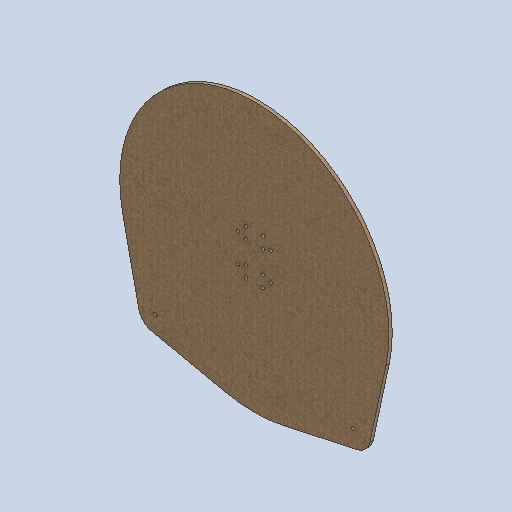
# Autodesk Inventor part: belt_liner_v1_MDF_throw_plate
Saved by Autodesk Inventor 2025.1 (Build 291241000, 241)
## iProperties
Created: 2024-12-08
Part Number: belt_liner_v1_MDF_throw_plate
Material: MDF 中密度繊維ボード
Document SubType Name: Modeling
Designer: haruy
Density: 0.8 g/cm^3
Appearance: ダンボール - 段ボール紙
Author: haruy
Autodesk Inventor part; units mm, degrees
ref_plane "YZ Plane" through (0, 0, 0) normal (1, 0, 0) x (0, 1, 0)
ref_plane "XZ Plane" through (0, 0, 0) normal (0, 1, 0) x (-1, 0, 0)
ref_plane "XY Plane" through (0, 0, 0) normal (0, 0, 1) x (1, 0, 0)
derived "belt_liner_v1_Sketch_Base.ipt"
sketch "スケッチ2" plane through (0, 0, 300) normal (0, 0, 1) x (1, 0, 0)
  circle A0 centre (0, 0) radius 120 projected
  circle A1 centre (-88.3883, -88.3883) radius 5 projected
  circle A2 centre (88.3883, -88.3883) radius 5 projected
  line L0 (0, 0) -> (0, -186.3039) projected
  line L1 (-10, 30) -> (10, 30) projected
  line L2 (10, 30) -> (10, -30) projected
  line L3 (10, -30) -> (-10, -30) projected
  line L4 (-10, -30) -> (-10, 30) projected
  line L5 (12, 2.5) -> (17, 2.5) projected
  line L6 (17, 2.5) -> (17, -2.5) projected
  line L7 (17, -2.5) -> (12, -2.5) projected
  line L8 (12, -2.5) -> (12, 2.5) projected
  circle A3 centre (-88.3883, -88.3883) radius 15 projected
  circle A4 centre (88.3883, -88.3883) radius 15 projected
  circle A5 centre (-7.5, -20) radius 1.5 projected
  circle A6 centre (-7.5, -10) radius 1.5 projected
  circle A7 centre (7.5, -10) radius 1.5 projected
  circle A8 centre (7.5, -20) radius 1.5 projected
  line L9 (0, 0) -> (10, 0) projected
  circle A9 centre (-7.5, 10) radius 1.5 projected
  circle A10 centre (-7.5, 20) radius 1.5 projected
  circle A11 centre (7.5, 10) radius 1.5 projected
  circle A12 centre (7.5, 20) radius 1.5 projected
  line L10 (12, 2.5) -> (17, 2.5) projected
  line L11 (17, 2.5) -> (17, 22.5) projected
  line L12 (17, 22.5) -> (12, 22.5) projected
  line L13 (12, 22.5) -> (12, 2.5) projected
  line L14 (12, -2.5) -> (17, -2.5) projected
  line L15 (17, -2.5) -> (17, -22.5) projected
  line L16 (17, -22.5) -> (12, -22.5) projected
  line L17 (12, -22.5) -> (12, -2.5) projected
  circle A13 centre (14.5, 12.5) radius 1.5 projected
  circle A14 centre (14.5, -12.5) radius 1.5 projected
  circle A15 centre (-14.5, 12.5) radius 1.5 projected
  circle A16 centre (-14.5, -12.5) radius 1.5 projected
  line L18 (-103.0529, -91.5429) -> (-117.3163, -25.2364) projected
  line L19 (-91.5429, -103.0529) -> (-25.2364, -117.3163) projected
  line L20 (91.5429, -103.0529) -> (25.2364, -117.3163) projected
  line L21 (103.0529, -91.5429) -> (117.3163, -25.2364) projected
  circle A17 centre (-88.3883, -88.3883) radius 1.5
  circle A18 centre (88.3883, -88.3883) radius 1.5
  point P0 (25.2364, -117.3163)
  dimension "d3" = 3
  dimension "d4" = 3
  constraints: 2 centre point, 2 coincident
  measures "d3" diameter of A17
  measures "d4" diameter of A18
extrude "押し出し1" add sketch "スケッチ2" against normal blind 3 contours A0 A4 A3 | A0 A3 L18 | L21 A4 A0 | A3 A0 | A1 | A0 A3 | A2 | A4 A0 | A0 A4 | A3 A0 L19 | A4 L20 A0 | L9 L2 L3 L0 | L0 L3 L4 L1 L2 L9 | L13 L12 L11 L5 | L5 L6 L7 L8 | L7 L15 L16 L17
